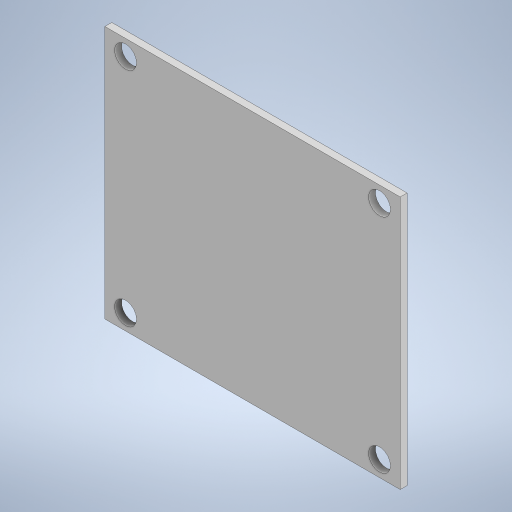
# Autodesk Inventor part: lcd 디스플레이
Saved by Autodesk Inventor 2023 (Build 270158000, 158)
## iProperties
Created: 2022-06-05
Part Number: lcd 디스플레이
Material: 일반
Document SubType Name: Modeling
Designer: fly01
Density: 1 g/cm^3
Appearance: 기본값
Author: fly01
Autodesk Inventor part; units mm, degrees
ref_plane "YZ Plane" through (0, 0, 0) normal (1, 0, 0) x (0, 1, 0)
ref_plane "XZ Plane" through (0, 0, 0) normal (0, 1, 0) x (-1, 0, 0)
ref_plane "XY Plane" through (0, 0, 0) normal (0, 0, 1) x (1, 0, 0)
sketch "스케치1" plane through (0, 0, 0) normal (0, 0, 1) x (1, 0, 0)
  line L0 (-42.7, 36.64) -> (42.7, 36.64)
  line L1 (42.7, 36.64) -> (42.7, -36.64)
  line L2 (42.7, -36.64) -> (-42.7, -36.64)
  line L3 (-42.7, -36.64) -> (-42.7, 36.64)
  line L4 (-42.7, 36.64) -> (42.7, -36.64) construction
  line L5 (42.7, 36.64) -> (-42.7, -36.64) construction
  circle A0 centre (36.72, 32.095) radius 3.1766
  line L6 (0, 0) -> (11.0996, 0) construction
  line L7 (0, 0) -> (0, 13.4158) construction
  circle A1 centre (-36.72, 32.095) radius 3.1766
  circle A2 centre (36.72, -32.095) radius 3.1766
  circle A3 centre (-36.72, -32.095) radius 3.1766
  dimension "d0" = 85.4
  dimension "d1" = 73.28
  dimension "d2" = 64.19
  dimension "d3" = 73.44
  constraints: 16 end point, 4 centre point, 3 symmetric about line, 2 horizontal, 2 midpoint, 2 parallel, 1 perpendicular, 1 vertical, 3 other
  measures "d0" distance of L1.end L2.end
  measures "d1" distance of L0.end L1.end
  measures "d2" distance of A2.centre A0.centre
  measures "d3" distance of A3.centre A2.centre
extrude "돌출1" add sketch "스케치1" along normal blind 2
